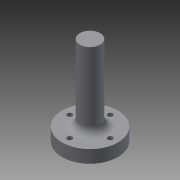
# Autodesk Inventor part: ax12tobase
Saved by Autodesk Inventor 2014 (Build 180170000, 170)
## iProperties
Created: 2014-01-13
Part Number: ax12tobase
Material: Générique
Document SubType Name: Modeling
Designer: helly
Density: 1 g/cm^3
Appearance: Par défaut
Author: helly
Autodesk Inventor part; units mm, degrees
ref_plane "YZ Plane" through (0, 0, 0) normal (1, 0, 0) x (0, 1, 0)
ref_plane "XZ Plane" through (0, 0, 0) normal (0, 1, 0) x (-1, 0, 0)
ref_plane "XY Plane" through (0, 0, 0) normal (0, 0, 1) x (1, 0, 0)
sketch "Esquisse1" plane through (0, 0, 0) normal (0, 0, 1) x (1, 0, 0)
  circle A0 centre (0, 0) radius 11
  circle A1 centre (0, 0) radius 8 construction
  line L0 (0, 0) -> (8, 0) construction
  circle A2 centre (8, 0) radius 1
  line L1 (0, 0) -> (0, 8) construction
  circle A3 centre (0, 8) radius 1
  line L2 (0, 0) -> (-8, 0) construction
  circle A4 centre (-8, 0) radius 1
  line L3 (0, 0) -> (0, -8) construction
  circle A5 centre (0, -8) radius 1
  dimension "d1" = 16
  dimension "d0" = 22
  dimension "d3" = 2
  dimension "d6" = 360
  constraints: 8 end point, 6 coincident, 5 centre point, 1 horizontal, 1 horizontal alignment, 23 other
  measures "d0" diameter of A0
  measures "d3" diameter of A2
extrude "Extrusion1" add sketch "Esquisse1" along normal blind 5
sketch "Esquisse2" plane through (0, 0, 5) normal (0, 0, 1) x (1, 0, 0)
  circle A0 centre (0, 0) radius 11 projected
  circle A1 centre (0, 0) radius 4
  dimension "d10" = 8
  constraints: 1 centre point, 1 coincident
  measures "d10" diameter of A1
extrude "Extrusion2" add sketch "Esquisse2" along normal blind 30 contours A1
sketch "Esquisse3" plane through (0, 0, 0) normal (0, 0, -1) x (-1, 0, 0)
  circle A0 centre (0, 0) radius 11 projected
  circle A1 centre (0, 0) radius 4
  dimension "d14" = 8
  constraints: 1 centre point, 1 coincident
  measures "d14" diameter of A1
extrude "Extrusion3" cut sketch "Esquisse3" against normal blind 1.5 contours A1
fillet "Congé1" radius 3 1 edges at (-4, 0, 5)
